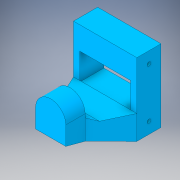
# Autodesk Inventor part: Carriage
Saved by Autodesk Inventor 2018.1 (Build 221171000, 171)
## iProperties
Created: 2017-12-03
Part Number: Carriage
Material: Generic
Document SubType Name: Modeling
Designer: xdlea
Density: 1 g/cm^3
Appearance: Default(1)
clothesHangerDia: 0.032 in
railWidth: 0.514 in
railHeight: 0.443 in
Author: xdlea
Autodesk Inventor part; units mm, degrees
ref_plane "YZ Plane" through (0, 0, 0) normal (1, 0, 0) x (0, 1, 0)
ref_plane "XZ Plane" through (0, 0, 0) normal (0, 1, 0) x (-1, 0, 0)
ref_plane "XY Plane" through (0, 0, 0) normal (0, 0, 1) x (1, 0, 0)
sketch "Sketch1" plane through (0, 0, 0) normal (0, 0, 1) x (1, 0, 0)
  line L0 (-0.35, 3.525) -> (13.05, 3.525)
  line L1 (13.05, 3.525) -> (13.05, -3.525)
  line L2 (13.05, -3.525) -> (-0.35, -3.525)
  line L3 (-0.35, -3.525) -> (-0.35, 3.525)
  line L4 (-1.9756, 9.525) -> (14.6756, 9.525)
  line L5 (14.6756, 9.525) -> (14.6756, -9.525)
  line L6 (14.6756, -9.525) -> (-1.9756, -9.525)
  line L7 (-1.9756, -9.525) -> (-1.9756, 9.525)
  circle A0 centre (6.35, 0) radius 2.3813 construction
  line L8 (0.2032, 3.175) -> (12.4968, 3.175) construction
  line L9 (12.7, 2.9718) -> (12.7, 2.2225) construction
  point P0 (0, 0)
  point P1 (6.35, 3.525)
  point P2 (6.35, 9.525)
  point P3 (13.05, 0)
  point P4 (14.6756, 0)
  dimension "d0" = 1.6256
  dimension "d1" = 19.05
  dimension "d2" = 0.35
  dimension "d3" = 0.35
  constraints: 16 end point, 4 midpoint, 4 parallel, 2 horizontal, 2 horizontal alignment, 2 perpendicular, 2 vertical alignment
  measures "d0" distance between parallel lines of L1 L5
  measures "d1" distance of L4.end L5.end
  measures "d2" distance between parallel lines of L1 L9
  measures "d3" distance between parallel lines of L8 L0
extrude "Extrusion1" add sketch "Sketch1" against normal blind 6.35
sketch "Sketch2" plane through (-1.9756, -9.525, 0) normal (0, -1, 0) x (1, 0, 0)
  line L0 (16.6512, 0) -> (0, 0) projected
  line L1 (0, 0) -> (4.3569, 9.2456)
  line L2 (4.3569, 9.2456) -> (4.3569, 14.3256)
  line L3 (4.3569, 14.3256) -> (12.2944, 14.3256)
  line L4 (12.2944, 14.3256) -> (12.2944, 9.2456)
  line L5 (12.2944, 9.2456) -> (16.6512, 0)
  line L6 (4.3569, 9.2456) -> (12.2944, 9.2456)
  line L7 (4.3569, 12.7) -> (12.2944, 12.7) construction
  line L8 (16.6512, -6.35) -> (0, -6.35) construction
  point P0 (1.9756, 0)
  point P1 (8.3256, 14.3256)
  point P2 (8.3256, 0)
  dimension "d6" = 7.9375
  dimension "d7" = 5.08
  dimension "d8" = 1.6256
  dimension "d9" = 19.05
  dimension "d21" = 14.3256
  constraints: 14 end point, 4 perpendicular, 2 midpoint, 2 point on line, 1 vertical, 1 vertical alignment
  measures "d6" distance of L2.end L3.end
  measures "d7" distance of L3.end L4.end
  measures "d8" distance between parallel lines of L7 L3
  measures "d9" distance between parallel lines of L7 L8
  measures "d21" distance between parallel lines of L0 L3
extrude "Extrusion2" add sketch "Sketch2" against normal blind 12.7 contours L6 L2 L3 L4
extrude "Extrusion3" add sketch "Sketch2" against normal blind 6.35 contours L0 L1 L6 L5
fillet "Fillet1" radius 3.9688 2 edges at (2.3812, 3.175, 11.7856) (10.3187, 3.175, 11.7856)
sketch "Sketch3" plane through (10.3187, -3.175, 9.2456) normal (0, 0, -1) x (-1, 0, 0)
  circle A0 centre (3.9688, 3.175) radius 2.3813 projected
  point P0 (10.3187, 3.175)
extrude "Extrusion4" cut sketch "Sketch3" against normal blind 3.4544
chamfer "Chamfer1" distance 14.3256 angle 15 1 edges at (6.35, -9.525, 14.3256) measured on face at (6.35, -9.525, 13.8256)
chamfer "Chamfer2" distance 2.54 angle 30 1 edges at (6.35, -3.175, 9.2456) measured on face at (6.35, -3.175, 8.7456)
sketch "Sketch4" plane through (-1.9756, -9.525, -6.35) normal (-1, 0, 0) x (0, 0, 1)
  circle A0 centre (3.175, 16.05) radius 0.4939
  circle A1 centre (3.175, 3) radius 0.4939
  line L0 (6.35, 13.05) -> (0, 13.05) construction
  line L1 (6.35, 13.05) -> (0, 13.05) projected
  line L2 (6.35, 19.05) -> (0, 19.05) construction
  line L3 (6.35, 19.05) -> (0, 19.05) projected
  line L4 (6.35, 19.05) -> (0, 19.05) construction
  line L5 (3.175, 19.05) -> (3.175, 13.05) construction
  line L6 (6.35, 13.05) -> (0, 13.05) construction
  line L7 (6.35, 9.525) -> (0, 9.525) construction
  line L8 (0, 0) -> (0, 19.05) construction
  line L9 (-8.078, 8.5123) -> (-8.078, 10.5377)
  point P0 (3.175, 16.05)
  dimension "d25" = 0.9878
  dimension "d28" = 13.05
  dimension "d29" = 11.253
  constraints: 6 end point, 4 midpoint, 2 centre point, 1 coincident, 1 equal radius, 1 symmetric about line, 1 vertical, 1 vertical alignment, 2 other
  measures "d25" diameter of A0
  measures "d28" distance of A1.centre A0.centre
  measures "d29" distance from line of A0.centre L9
extrude "Extrusion5" cut sketch "Sketch4" against normal up to next
equation "\"d14\" = 0.5 * d6"
equation "\"d15\" = d7 - d8"
equation "\"d17\" = d21"
equation "\"d26\" = d7 - d8"
equation "\"clothesHangerDia\" = 0.8128"
equation "\"railWidth\" = d28"
equation "\"railHeight\" = d29"
body "Solid1"
